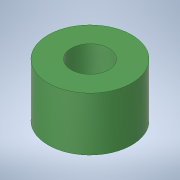
# Autodesk Inventor part: 071_0105_ScrewCap
Saved by Autodesk Inventor 2020 (Build 240168000, 168)
## iProperties
Created: 2018-12-03
Part Number: 071_0105_ScrewCap
Material: Generic
Document SubType Name: Modeling
Designer: Gio
Density: 1 g/cm^3
Appearance: Default
Author: Gio
Autodesk Inventor part; units mm, degrees
ref_plane "YZ Plane" through (0, 0, 0) normal (1, 0, 0) x (0, 1, 0)
ref_plane "XZ Plane" through (0, 0, 0) normal (0, 1, 0) x (-1, 0, 0)
ref_plane "XY Plane" through (0, 0, 0) normal (0, 0, 1) x (1, 0, 0)
sketch "Sketch1" plane through (0, 0, 0) normal (0, 1, 0) x (-1, 0, 0)
  circle A0 centre (0, 0) radius 5.45
  dimension "d0" = 10.9
  constraints: 1 centre point, 1 coincident
  measures "d0" diameter of A0
extrude "Extrusion1" add sketch "Sketch1" along normal blind 7
shell "Shell1" thickness 3 removed faces 1 at (-1.7639, 7, -0.4348)
equation "\"d0\" = screw_diameter + 2 * thickness"
equation "\"d1\" = height + thickness"
equation "\"d3\" = thickness"
equation "\"screw_diameter\" = 4.9"
equation "\"thickness\" = 3"
equation "\"height\" = 4"
body "Solid1"
